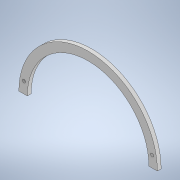
# Autodesk Inventor part: Montage_Ring_Hinten_Teil1
Saved by Autodesk Inventor 2022.2 (Build 262287010, 287A)
## iProperties
Created: 2024-01-10
Part Number: Montage_Ring_Hinten_Teil1
Material: Generisch
Document SubType Name: Modeling
Designer: ppovolni
Density: 1 g/cm^3
Appearance: Vorgabe
Author: ppovolni
Autodesk Inventor part; units mm, degrees
ref_plane "YZ Plane" through (0, 0, 0) normal (1, 0, 0) x (0, 1, 0)
ref_plane "XZ Plane" through (0, 0, 0) normal (0, 1, 0) x (-1, 0, 0)
ref_plane "XY Plane" through (0, 0, 0) normal (0, 0, 1) x (1, 0, 0)
sketch "Skizze1" plane through (0, 0, 0) normal (0, 0, 1) x (1, 0, 0)
  circle A0 centre (0, 0) radius 80.1 construction
  circle A1 centre (0, 0) radius 93.8 construction
  circle A2 centre (0, 0) radius 80.6
  circle A3 centre (0, 0) radius 91.8
  line L0 (-91.8, 0) -> (-80.6, 0)
  line L1 (80.6, 0) -> (91.8, 0)
  circle A4 centre (0, 0) radius 86.2 construction
  circle A5 centre (-84.8904, 14.9685) radius 2.05
  circle A6 centre (84.8904, 14.9685) radius 2.05
  line L2 (0, 0) -> (-84.8904, 14.9685) construction
  line L3 (0, 0) -> (84.8904, 14.9685) construction
  point P0 (0, 86.1)
  point P1 (5.5, 80.4121)
  point P2 (-5.5, 80.4121)
  dimension "d0" = 160.2
  dimension "d1" = 187.6
  dimension "d2" = 0.5
  dimension "d3" = 2
  dimension "d8" = 5.6
  dimension "d9" = 4.1
  dimension "d10" = 10
  dimension "d11" = 10
  constraints: 8 end point, 8 point on circle, 7 centre point, 5 coincident, 2 point on line, 1 equal radius, 1 vertical alignment
  measures "d0" diameter of A0
  measures "d1" diameter of A1
  measures "d2" radial gap between concentric circles of A0 A2
  measures "d3" radial gap between concentric circles of A3 A1
  measures "d8" radial gap between concentric circles of A4 A3
  measures "d9" diameter of A5
  measures "d10" angle of L1 L3
  measures "d11" angle of L0 L2
extrude "Extrusion1" add sketch "Skizze1" along normal blind 5 contours A2 L0 A3 L1 picked at (4.3548, 87.7552)
